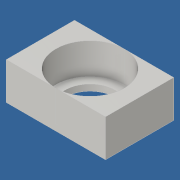
# Autodesk Inventor part: rotSpanner
Saved by Autodesk Inventor 2016 (Build 200138000, 138)
## iProperties
Created: 2016-03-28
Part Number: rotSpanner
Material: ABS-Kunststoff
Document SubType Name: Modeling
Designer: 4ndreas
Density: 1.06 g/cm^3
Appearance: Glatt - weiß
Mass: 0.562403 g
Surface Area: 7.73389 cm^2
Volume: 0.530569 cm^3
Author: 4ndreas
Autodesk Inventor part; units mm, degrees
ref_plane "YZ Plane" through (0, 0, 0) normal (1, 0, 0) x (0, 1, 0)
ref_plane "XZ Plane" through (0, 0, 0) normal (0, 1, 0) x (-1, 0, 0)
ref_plane "XY Plane" through (0, 0, 0) normal (0, 0, 1) x (1, 0, 0)
sketch "Skizze1" plane through (0, 0, 0) normal (0, 0, 1) x (1, 0, 0)
  line L0 (-8, -5.5) -> (8, -5.5)
  line L1 (8, -5.5) -> (8, 5.5)
  line L2 (8, 5.5) -> (-8, 5.5)
  line L3 (-8, 5.5) -> (-8, -5.5)
  line L4 (-8, -5.5) -> (8, 5.5) construction
  line L5 (8, -5.5) -> (-8, 5.5) construction
  circle A0 centre (0, 0) radius 5.5
  circle A1 centre (0, 0) radius 4
  dimension "d0" = 11
  dimension "d1" = 16
  dimension "d6" = 8
  constraints: 12 end point, 2 centre point, 2 coincident, 2 midpoint, 2 parallel, 1 horizontal, 1 perpendicular, 1 tangent
  measures "d0" diameter of A0
  measures "d1" distance between parallel lines of L1 L3
  measures "d6" diameter of A1
extrude "Extrusion1" add sketch "Skizze1" along normal blind 5 contours L3 L2 A0 L0 | A0 L2 L1 L0
extrude "Extrusion2" add sketch "Skizze1" against normal blind 1 contours L3 L2 A0 L0 | A0 L2 L1 L0 | A0 | A1
extrude "Extrusion3" cut sketch "Skizze1" against normal through all contours A1
